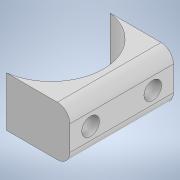
# Autodesk Inventor part: CatchHolderNut
Saved by Autodesk Inventor 2020 (Build 240168000, 168)
## iProperties
Created: 2022-01-23
Part Number: CatchHolderNut
Material: Generic
Document SubType Name: Modeling
Designer: pab2
Density: 1 g/cm^3
Appearance: Default
Author: pab2
Autodesk Inventor part; units mm, degrees
ref_plane "YZ Plane" through (0, 0, 0) normal (1, 0, 0) x (0, 1, 0)
ref_plane "XZ Plane" through (0, 0, 0) normal (0, 1, 0) x (-1, 0, 0)
ref_plane "XY Plane" through (0, 0, 0) normal (0, 0, 1) x (1, 0, 0)
sketch "Sketch1" plane through (0, 0, 0) normal (0, 1, 0) x (-1, 0, 0)
  line L0 (0, 0) -> (26.416, 0)
  line L1 (26.416, 0) -> (26.416, -26.416)
  line L2 (26.416, -26.416) -> (0, -26.416)
  line L3 (0, -26.416) -> (0, 0)
  line L4 (0, -13.208) -> (17.9832, -13.208)
  line L5 (0, -13.208) -> (17.9832, -13.208) construction
  circle A0 centre (17.9832, -13.208) radius 13.335
  point P0 (16.1472, 0)
  point P1 (16.1472, -26.416)
  dimension "d0" = 26.416
  dimension "d1" = 26.416
  dimension "d2" = 17.9832
  dimension "d3" = 0
  dimension "d4" = 26.67
  constraints: 12 end point, 3 horizontal, 2 parallel, 1 centre point, 1 coincident, 1 collinear, 1 midpoint, 1 perpendicular
  measures "d0" distance of L1.end L2.end
  measures "d1" distance of L0.end L1.end
  measures "d2" distance of L4.start L4.end
  measures "d3" distance between parallel lines of L4 L5
  measures "d4" diameter of A0
extrude "Extrusion1" add sketch "Sketch1" along normal blind 12.7 contours L0 A0 L4 L3 | L4 A0 L2 L3
sketch "Sketch2" plane through (0, 0, 0) normal (1, 0, 0) x (0, 0, -1)
  line L0 (0, 12.7) -> (26.416, 12.7) projected
  line L1 (13.208, 12.7) -> (13.208, 6.35)
  line L2 (13.208, 12.7) -> (19.558, 12.7) construction
  line L3 (13.208, 6.35) -> (21.1328, 6.35)
  line L4 (13.208, 6.35) -> (21.1328, 6.35) construction
  line L5 (13.208, 6.35) -> (5.2832, 6.35)
  line L6 (13.208, 6.35) -> (21.1328, 6.35) construction
  point P0 (0, 0)
  dimension "d7" = 6.35
  dimension "d8" = 90
  dimension "d9" = 7.9248
  dimension "d10" = 0
  dimension "d11" = 7.9248
  dimension "d12" = 180
  constraints: 12 end point, 5 horizontal, 3 equal length, 1 midpoint, 1 vertical
  measures "d7" distance of L1.start L1.end
  measures "d8" angle of L1 L2
  measures "d9" distance of L1.end L3.end
  measures "d10" distance between parallel lines of L3 L4
  measures "d11" distance of L1.end L5.end
  measures "d12" angle of L5 L6
hole "Hole1" at (0, 6.35, -5.2832) at (0, 6.35, -21.1328) direction (-1, 0, 0) diameter 4.4958 depth 35 start extended yes clearance for "Flat Head Machine Screw (82)" size "#8" standard "Ansi Unified Screw Threads"
fillet "Fillet1" radius 3.175 2 edges at (0, 12.7, -13.208) (0, 0, -13.208)
body "Solid1"
